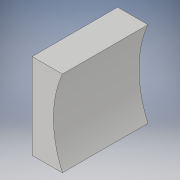
# Autodesk Inventor part: Air Cylinder Wood Mounting Block
Saved by Autodesk Inventor 2018.3 (Build 223284000, 284)
## iProperties
Created: 2019-03-03
Part Number: Air Cylinder Wood Mounting Block
Material: Generic
Document SubType Name: Modeling
Designer: Refraction
Density: 1 g/cm^3
Appearance: Default
Author: Refraction
Autodesk Inventor part; units mm, degrees
ref_plane "YZ Plane" through (0, 0, 0) normal (1, 0, 0) x (0, 1, 0)
ref_plane "XZ Plane" through (0, 0, 0) normal (0, 1, 0) x (-1, 0, 0)
ref_plane "XY Plane" through (0, 0, 0) normal (0, 0, 1) x (1, 0, 0)
sketch "Sketch1" plane through (0, 0, 0) normal (0, 0, 1) x (1, 0, 0)
  line L0 (0, 0) -> (38.1, 0)
  line L1 (38.1, 0) -> (38.1, 25.4)
  line L2 (38.1, 25.4) -> (0, 25.4)
  line L3 (0, 25.4) -> (0, 0)
  line L4 (38.1, 12.7) -> (6.35, 12.7) construction
  circle A0 centre (38.1, 12.7) radius 31.75
  dimension "d0" = 38.1
  dimension "d1" = 25.4
  dimension "d2" = 31.75
  constraints: 10 end point, 2 horizontal, 2 parallel, 1 coincident, 1 horizontal alignment, 1 midpoint, 1 perpendicular, 2 other
  measures "d0" distance of L2.end L1.end
  measures "d1" distance of L1.end L0.end
  measures "d2" distance of L4.start L4.end
extrude "Extrusion1" add sketch "Sketch1" along normal blind 25.4 contours L3 L2 A0 L0 | A0 L2 L1 L0 picked at (27.5167, 12.7)
sketch "Sketch2" plane through (0, 0, 25.4) normal (0, 0, 1) x (1, 0, 0)
  line L0 (38.1, 0) -> (38.1, 25.4) construction
  line L1 (38.1, 12.7) -> (6.35, 12.7) construction
  circle A0 centre (38.1, 12.7) radius 31.75
  point P0 (0, 0)
  dimension "d5" = 31.75
  constraints: 2 end point, 1 coincident, 1 horizontal, 1 horizontal alignment, 1 midpoint, 2 other
  measures "d5" distance of L1.start L1.end
extrude "Extrusion2" cut sketch "Sketch2" against normal blind 25.4
body "Solid1"
